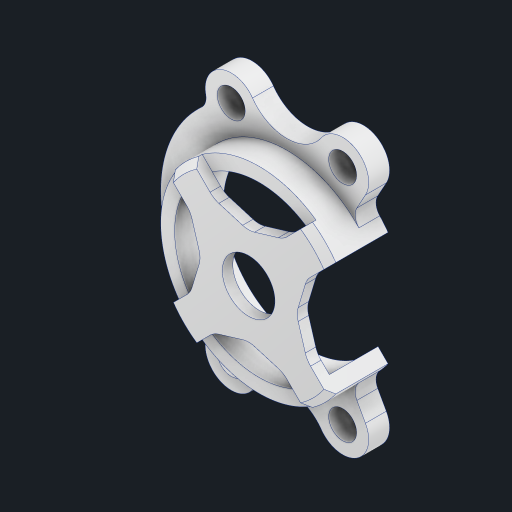
# Autodesk Inventor part: PotentiometerCover
Saved by Autodesk Inventor 2023 (Build 270158000, 158)
## iProperties
Created: 2023-07-17
Part Number: PotentiometerCover
Material: Aluminum 6061
Document SubType Name: Modeling
Designer: valer
Density: 2.7 g/cm^3
Appearance: Aluminum - Flat
Author: valer
Autodesk Inventor part; units mm, degrees
ref_plane "YZ Plane" through (0, 0, 0) normal (1, 0, 0) x (0, 1, 0)
ref_plane "XZ Plane" through (0, 0, 0) normal (0, 1, 0) x (-1, 0, 0)
ref_plane "XY Plane" through (0, 0, 0) normal (0, 0, 1) x (1, 0, 0)
sketch "Base" plane through (0, 0, 0) normal (0, 0, 1) x (1, 0, 0)
  arc A0 (-3.005734, -11.807241) -> (-3.005734, -19.807241) centre (-14.319443, -15.807241) ccw construction
  circle A1 centre (-14.319443, -15.807241) radius 3.775
  circle A2 centre (-14.319443, -15.807241) radius 12.125
  circle A3 centre (-14.319443, -15.807241) radius 14.125
  point P0 (0, 0)
  dimension "d1" = 12
  dimension "d2" = 24.25
  dimension "d3" = 2
  constraints: 2 centre point, 2 coincident
  measures "d1" radius of A0
  measures "d2" diameter of A2
  measures "d3" radial gap between concentric circles of A2 A3
extrude "BaseFeature" add sketch "Base" along normal blind 1.5 contours A2 | A3
sketch "Head" plane through (-14.319443, -15.807241, 0) normal (0, 0, -1) x (-1, 0, 0)
  circle A0 centre (0, 0) radius 14.125 projected
  circle A1 centre (0, 0) radius 12.125 projected
  point P0 (-14.319443, 15.807241)
extrude "HeadFeature" add sketch "Head" along normal blind 7
sketch "Mount" plane through (-14.319443, -15.807241, -7) normal (0, 0, -1) x (-1, 0, 0)
  line L0 (-24, 24) -> (24, 24) construction
  line L1 (24, 24) -> (24, -24) construction
  line L2 (24, -24) -> (-24, -24) construction
  line L3 (-24, -24) -> (-24, 24) construction
  line L4 (0, 24) -> (0, -24) construction
  line L5 (-24, 0) -> (24, 0) construction
  circle A0 centre (0, 0) radius 7
  circle A1 centre (0, 0) radius 12 construction
  line L6 (0, 12) -> (-12, 0) construction
  line L7 (-12, 0) -> (0, -12) construction
  line L8 (0, -12) -> (12, 0) construction
  line L9 (12, 0) -> (0, 12) construction
  line L10 (-24, 16) -> (24, 16) construction
  line L11 (-24, 8) -> (24, 8) construction
  line L12 (-24, -8) -> (24, -8) construction
  line L13 (-24, -16) -> (24, -16) construction
  line L14 (-16, 24) -> (-16, -24) construction
  line L15 (-8, 24) -> (-8, -24) construction
  line L16 (16, 24) -> (16, -24) construction
  line L17 (8, 24) -> (8, -24) construction
  circle A2 centre (-8, 16) radius 2
  circle A3 centre (-16, 8) radius 2 construction
  circle A4 centre (8, 16) radius 2
  line L18 (24, 8) -> (-24, 8) construction
  circle A5 centre (16, 8) radius 2 construction
  circle A6 centre (-16, -8) radius 2 construction
  circle A7 centre (-8, -16) radius 2
  circle A8 centre (8, -16) radius 2
  circle A9 centre (16, -8) radius 2 construction
  circle A10 centre (0, 0) radius 14.125 projected
  circle A11 centre (0, 0) radius 21.625
  circle A12 centre (0, 0) radius 14.125 projected
  point P0 (-14.319443, 15.807241)
  dimension "d8" = 14
  dimension "d9" = 24
  dimension "d10" = 48
  dimension "d11" = 8
  dimension "d12" = 8
  dimension "d13" = 8
  dimension "d14" = 8
  dimension "d40" = 7.5
  constraints: 38 end point, 16 symmetric about line, 14 point on line, 11 centre point, 8 perpendicular, 5 midpoint, 4 coincident, 4 parallel, 2 point on circle, 1 horizontal, 6 other
  measures "d8" diameter of A0
  measures "d9" diameter of A1
  measures "d10" distance of L3.end L0.end
  measures "d11" distance between parallel lines of L0 L10
  measures "d12" distance between parallel lines of L11 L10
  measures "d13" distance between parallel lines of L3 L14
  measures "d14" distance between parallel lines of L14 L15
  measures "d40" radial gap between concentric circles of A11 A12
extrude "MountFeature" add sketch "Mount" against normal blind 3 contours A11
sketch "Cuts" plane through (-14.319443, -15.807241, 1.5) normal (0, 0, 1) x (1, 0, 0)
  circle A0 centre (0, 0) radius 14.125
  line L0 (-11.523905, -8.16794) -> (-8.355965, -5)
  line L1 (-8.355965, -5) -> (-8.355965, 5) construction
  line L2 (-8.355965, 5) -> (-11.523905, 8.16794)
  line L3 (-8.355965, 0) -> (-14.125, 0) construction
  line L4 (0, 0) -> (-21.625, 0) construction
  circle A1 centre (0, 0) radius 21.625
  line L5 (0, 0) -> (0, -21.625) construction
  line L6 (-5, -8.355965) -> (-8.16794, -11.523905)
  line L7 (-8.16794, -11.523905) -> (-11.523905, -8.16794) construction
  line L8 (0, 0) -> (-15.291184, -15.291184) construction
  circle A2 centre (-8, -16) radius 2 construction
  circle A3 centre (-16, -8) radius 2 construction
  line L9 (-8, -16) -> (-16, -8) construction
  line L10 (-5, -8.355965) -> (-8.355965, -5) construction
  line L11 (-5, 8.355965) -> (-8.16794, 11.523905)
  line L12 (-8.355965, -5) -> (-6.855965, 0)
  line L13 (-8.355965, 5) -> (-6.855965, 0)
  line L14 (11.523905, -8.16794) -> (8.355965, -5)
  line L15 (8.355965, -5) -> (8.355965, 5) construction
  line L16 (8.355965, 5) -> (11.523905, 8.16794)
  line L17 (5, -8.355965) -> (8.16794, -11.523905)
  line L18 (5, -8.355965) -> (8.355965, -5) construction
  line L19 (5, 8.355965) -> (8.16794, 11.523905)
  line L20 (8.355965, -5) -> (6.855965, 0)
  line L21 (8.355965, 5) -> (6.855965, 0)
  line L22 (5, -8.355965) -> (-5, -8.355965) construction
  line L23 (5, 8.355965) -> (-5, 8.355965) construction
  line L24 (5, -8.355965) -> (0, -6.855965)
  line L25 (-5, -8.355965) -> (0, -6.855965)
  line L26 (5, 8.355965) -> (0, 6.855965)
  line L27 (0, 6.855965) -> (-5, 8.355965)
  circle A4 centre (16, -8) radius 2 construction
  circle A5 centre (16, 8) radius 2 construction
  point P0 (14.319443, 15.807241)
  point P1 (-12, -12)
  point P2 (-6.677982, -6.677982)
  point P3 (8.16794, 11.523905)
  point P4 (-8.16794, 11.523905)
  point P5 (8.16794, -11.523905)
  point P6 (11.523905, -8.16794)
  point P7 (11.523905, 8.16794)
  dimension "d20" = 45
  dimension "d22" = 45
  dimension "d23" = 10
  dimension "d24" = 45
  dimension "d26" = 1.5
  dimension "d27" = 1.5
  dimension "d28" = 1.5
  constraints: 56 end point, 13 symmetric about line, 7 point on circle, 4 horizontal, 4 point on line, 3 centre point, 3 midpoint, 2 vertical, 1 collinear, 1 equal length, 1 perpendicular, 3 other
  measures "d20" angle of L3 L2
  measures "d22" angle of L0 L3
  measures "d23" distance of L0.end L1.end
  measures "d24" angle of L6 L5
  measures "d26" distance from line of L1 L12.end
  measures "d27" distance from line of L22 L24.end
  measures "d28" distance from line of L23 L26.end
extrude "CutsFeature" cut sketch "Cuts" against normal blind 1.5 contours A0 L14 L20 L21 L16 | L19 L26 L27 L11 A0 | A0 L6 L25 L24 L17 | L2 L13 L12 L0 A0
chamfer "CutsChamferFeature" distance 1 angle 45 4 edges at (-4.3316, -5.8194, 1.5) (-4.3316, -25.7951, 1.5) (-24.3073, -5.8194, 1.5) (-24.3073, -25.7951, 1.5)
fillet "CutsFilletFeature" radius 3 12 edges at (-5.9635, -10.8072, 0.75) (-7.4635, -15.8072, 0.75) (-5.9635, -20.8072, 0.75) (-22.6754, -10.8072, 0.75) (-21.1754, -15.8072, 0.75) (-22.6754, -20.8072, 0.75) (-19.3194, -24.1632, 0.75) (-14.3194, -22.6632, 0.75) (-9.3194, -24.1632, 0.75) (-19.3194, -7.4513, 0.75) (-14.3194, -8.9513, 0.75) (-9.3194, -7.4513, 0.75)
sketch "LeadCut" plane through (-14.319443, -15.807241, 0) normal (0, 0, 1) x (1, 0, 0)
  line L0 (11.046068, -5) -> (14.125, -5)
  line L1 (14.125, -5) -> (14.125, 5)
  line L2 (14.125, 5) -> (11.046068, 5)
  line L3 (11.046068, 5) -> (11.046068, -5)
  line L4 (0, 0) -> (21.625, 0) construction
  circle A0 centre (0, 0) radius 21.625
  arc A1 (10.085847, -6.729882) -> (10.085847, 6.729882) centre (0, 0) ccw construction
  arc A2 (11.523905, -8.16794) -> (11.523905, 8.16794) centre (0, 0) ccw construction
  circle A3 centre (0, 0) radius 3.775
  line L5 (0, 0) -> (0, 21.625) construction
  point P0 (14.319443, 15.807241)
  point P1 (14.125, 0)
  dimension "d35" = 10
  constraints: 12 end point, 4 point on circle, 2 horizontal, 2 parallel, 1 coincident, 1 midpoint, 1 perpendicular, 1 point on line, 1 vertical
  measures "d35" distance of L0.end L1.end
extrude "LeadCutFeature" cut sketch "LeadCut" against normal up to surface (4 mm away) contours L3 L2 L1 L0
sketch "Sketch10" plane through (-14.319443, -15.807241, 0) normal (0, 0, 1) x (1, 0, 0)
  line L0 (13.210436, -5) -> (11.046068, -5)
  arc A0 (10.085847, -6.729882) -> (11.046068, -5) centre (0, 0) ccw
  line L1 (11.523905, -8.16794) -> (10.085847, -6.729882)
  arc A1 (11.523905, -8.16794) -> (13.210436, -5) centre (0, 0) ccw
  line L2 (11.046068, 5) -> (13.210436, 5)
  arc A2 (13.210436, 5) -> (11.523905, 8.16794) centre (0, 0) ccw
  line L3 (10.085847, 6.729882) -> (11.523905, 8.16794)
  arc A3 (11.046068, 5) -> (10.085847, 6.729882) centre (0, 0) ccw
  point P0 (14.319443, 15.807241)
extrude "Extrusion7" cut sketch "Sketch10" against normal up to surface (4 mm away)
sketch "MountProfile" plane through (-14.319443, -15.807241, -4) normal (0, 0, 1) x (1, 0, 0)
  circle A0 centre (8, 16) radius 2
  circle A1 centre (0, 0) radius 3.775
  line L0 (0, 0.123127) -> (-15.291184, 15.291184) construction
  line L1 (0, 0.123127) -> (0, 21.7) construction
  circle A2 centre (-8, 16) radius 2
  arc A3 (11.046068, -5) -> (11.046068, 5) centre (0, 0) ccw
  arc A4 (-11.271146, 14.194256) -> (-11.271146, -14.194256) centre (0, 0) ccw
  arc A5 (10.085847, -6.729882) -> (10.085847, 6.729882) centre (0, 0) ccw
  arc A6 (8.16794, -11.523905) -> (11.523905, -8.16794) centre (0, 0) ccw
  line L2 (11.523905, 8.16794) -> (10.085847, 6.729882)
  line L3 (11.523905, -8.16794) -> (10.804876, -7.448911) construction
  line L4 (10.085847, -6.729882) -> (11.523905, -8.16794)
  arc A7 (11.523905, 8.16794) -> (8.16794, 11.523905) centre (0, 0) ccw
  line L5 (8.890787, 5.534822) -> (10.805807, 7.449843)
  line L6 (10.805807, 7.449843) -> (11.523905, 8.16794)
  line L7 (10.805807, -7.449843) -> (8.890787, -5.534822)
  arc A8 (11.523905, 8.16794) -> (11.523905, -8.16794) centre (0, 0) ccw
  circle A9 centre (0, 0) radius 21.625
  circle A10 centre (-8, -16) radius 2
  circle A11 centre (-8, -16) radius 2
  circle A12 centre (-8, -16) radius 3.736456
  circle A13 centre (0, 0) radius 21.625
  circle A14 centre (0, -21.625) radius 6.043146
  arc A15 (11.271146, -14.194256) -> (11.271146, 14.194256) centre (0, 0) ccw
  circle A16 centre (8, -16) radius 3.736456
  line L8 (-21.625, 0) -> (0, 0) construction
  circle A17 centre (-8, 16) radius 3.736456
  circle A18 centre (0, 21.625) radius 6.043146
  circle A19 centre (8, 16) radius 3.736456
  line L9 (11.271146, 14.194256) -> (9.302929, 10.628788)
  line L10 (11.271146, -14.194256) -> (9.302929, -10.628788)
  point P0 (-11.128342, 5)
  point P1 (-11.128342, -5)
  point P2 (11.046068, 5)
  point P3 (11.046068, -5)
  point P4 (11.271146, 14.194256)
  point P5 (9.670994, -19.341988)
  point P6 (9.670994, 19.341988)
  point P7 (-9.670994, 19.341988)
  point P8 (-4.94347, 18.149123)
  point P9 (4.94347, 18.149123)
  point P10 (-9.670994, -19.341988)
  point P11 (-4.94347, -18.149123)
  point P12 (4.94347, -18.149123)
  dimension "d47" = 4
  constraints: 12 end point, 7 point on circle, 7 symmetric about line, 5 centre point, 2 horizontal, 2 vertical, 1 coincident, 1 midpoint, 1 tangent, 16 other
  measures "d47" radial gap between concentric circles of A8 A4
extrude "MountProfileFeature" cut sketch "MountProfile" against normal through all contours A0 | A2 | A3 A5 L2 A7 L9 A15 L10 A6 L4 | A15 A19 A9 A16 | A16 A9 A14 | A14 A9 | A18 A9 | A18 A9 A19 | A14 A9 A12 | A17 A9 A18 | A9 A17 A4 A12 picked at (0, -19.547706) picked at (0, 19.547706)
fillet "Fillet2" radius 2 4 edges at (-25.5906, -30.0015, -5.5) (-25.5906, -1.613, -5.5) (-5.0165, -26.436, -5.5) (-5.0165, -5.1785, -5.5)
equation "\"d22\" = d20"
equation "\"d24\" = d20"
equation "\"d27\" = d26"
equation "\"d28\" = d26"
body "Solid1"
